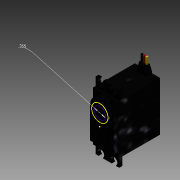
# Autodesk Inventor part: Tetrix 180 Servo
Saved by Autodesk Inventor 2013 (Build 170138000, 138)
## iProperties
Created: 2012-11-17
Part Number: Tetrix 180 Servo
Material: Generic
Document SubType Name: Modeling
Designer: niemitalo_dan
Density: 1 g/cm^3
Author: niemitalo_dan
Autodesk Inventor part; units mm, degrees
ref_plane "YZ Plane" through (0, 0, 0) normal (1, 0, 0) x (0, 1, 0)
ref_plane "XZ Plane" through (0, 0, 0) normal (0, 1, 0) x (-1, 0, 0)
sketch "Hole Pattern 4" plane through (0, 0, 0) normal (0, 0, 1) x (1, 0, 0)
  circle A0 centre (-145.7144, 104.3642) radius 4
  circle A1 centre (-145.7144, 104.3642) radius 8 construction
  circle A2 centre (-145.7144, 112.3642) radius 1.85
  circle A3 centre (-145.7144, 96.3642) radius 1.85
  circle A4 centre (-153.7144, 104.3642) radius 1.85
  circle A5 centre (-137.7144, 104.3642) radius 1.85
  circle A6 centre (-145.7144, 120.3642) radius 4
  circle A7 centre (-145.7144, 88.3642) radius 4
  point P0 (-145.7144, 107.7928)
  dimension "d140" = 16
  dimension "d141" = 3.7
  dimension "d142" = 16
  dimension "d143" = 16
  dimension "d144" = 8
  measures "d140" diameter of A1
  measures "d141" diameter of A2
  measures "d142" distance of A6.centre A0.centre
  measures "d143" distance of A7.centre A0.centre
  measures "d144" diameter of A0
sketch "Sketch1" plane through (0, 0, 0) normal (0, 0, 1) x (1, 0, 0)
  line L0 (-9.9314, 19.3675) -> (9.9314, 19.3675)
  line L1 (9.9314, 19.3675) -> (9.9314, -19.3675)
  line L2 (9.9314, -19.3675) -> (-9.9314, -19.3675)
  line L3 (-9.9314, -19.3675) -> (-9.9314, 19.3675)
  point P0 (0, 0)
  point P1 (-9.9314, 0)
  point P2 (0, 19.3675)
  dimension "d0" = 19.8628
  dimension "d1" = 38.735
  constraints: 8 end point, 2 midpoint, 2 parallel, 1 horizontal, 1 horizontal alignment, 1 perpendicular, 1 vertical alignment
  measures "d0" distance of L1.end L2.end
  measures "d1" distance of L0.end L1.end
extrude "Extrusion1" add sketch "Sketch1" along normal blind 33.147
sketch "Sketch2" plane through (0, 0, 33.147) normal (0, 0, 1) x (1, 0, 0)
  line L0 (9.9314, 19.3675) -> (-9.9314, 19.3675) projected
  line L1 (-9.9314, 19.3675) -> (-9.9314, -19.3675) projected
  line L2 (-9.9314, -19.3675) -> (9.9314, -19.3675) projected
  line L3 (-9.2964, 18.7325) -> (9.2964, 18.7325)
  line L4 (9.2964, 18.7325) -> (9.2964, -15.0495)
  line L5 (9.2964, -15.0495) -> (-9.2964, -15.0495)
  line L6 (-9.2964, -15.0495) -> (-9.2964, 18.7325)
  arc A0 (-3.6998, -15.0495) -> (3.6998, -15.0495) centre (0, -10.9617) ccw
  point P0 (0, 0)
  point P1 (0, 18.7325)
  dimension "d4" = 0.635
  dimension "d5" = 0.635
  dimension "d6" = 4.318
  constraints: 8 end point, 2 parallel, 2 point on circle, 2 point on line, 2 vertical alignment, 1 centre point, 1 horizontal, 1 midpoint, 1 perpendicular
  measures "d4" distance between parallel lines of L0 L3
  measures "d5" distance between parallel lines of L1 L6
  measures "d6" distance between parallel lines of L2 L5
extrude "Extrusion2" add sketch "Sketch2" along normal blind 2.794 contours L3 L4 L5 L6
sketch "Sketch3" plane through (0, 0, 35.941) normal (0, 0, 1) x (1, 0, 0)
  circle A0 centre (0, 9.4361) radius 6.4516
  line L0 (9.9314, 19.3675) -> (-9.9314, 19.3675) projected
  point P0 (0, 0)
  dimension "d9" = 12.9032
  dimension "d11" = 9.9314
  constraints: 1 centre point, 1 vertical alignment
  measures "d9" diameter of A0
  measures "d11" distance from line of L0 A0.centre
extrude "Extrusion3" add sketch "Sketch3" along normal blind 1.778
fillet "Fillet1" radius 9.2964 2 edges at (9.2964, 18.7325, 34.544) (-9.2964, 18.7325, 34.544)
ref_plane "Work Plane1" through (0, 0, 29.083) normal (0, 0, 1) x (1, 0, 0)
sketch "Sketch4" plane through (0, 0, 29.083) normal (0, 0, 1) x (1, 0, 0)
  line L0 (9.9314, 19.3675) -> (9.9314, -19.3675) projected
  line L1 (9.9314, -19.3675) -> (-9.9314, -19.3675) projected
  line L2 (-9.9314, -19.3675) -> (-9.9314, 19.3675) projected
  line L3 (-9.9314, 19.3675) -> (9.9314, 19.3675) projected
  line L4 (-9.3599, 19.3675) -> (9.3599, 19.3675)
  line L5 (9.3599, 19.3675) -> (9.3599, 26.4795)
  line L6 (-9.3599, 26.4795) -> (-9.3599, 19.3675)
  circle A0 centre (-5.1689, 23.9395) radius 2.667
  circle A1 centre (5.1689, 23.9395) radius 2.667
  line L7 (-5.9821, 26.4795) -> (-9.3599, 26.4795)
  line L8 (9.3599, 26.4795) -> (5.9821, 26.4795)
  line L9 (4.3557, 26.4795) -> (-4.3557, 26.4795)
  point P0 (0, 0)
  point P1 (0, 26.4795)
  dimension "d16" = 18.7198
  dimension "d18" = 7.112
  dimension "d20" = 5.334
  dimension "d21" = 4.191
  dimension "d22" = 4.191
  constraints: 12 end point, 4 parallel, 4 point on circle, 2 centre point, 1 equal radius, 1 horizontal, 1 horizontal alignment, 1 midpoint, 1 perpendicular, 1 point on line, 1 vertical alignment
  measures "d16" distance of L5.end L6.start
  measures "d18" distance of L6.start L4.start
  measures "d20" diameter of A0
  measures "d21" distance from line of L6 A0.centre
  measures "d22" distance from line of L5 A1.centre
extrude "Extrusion4" add sketch "Sketch4" along normal blind 2.54 contours L3 L6 L7 A0 L9 A1 L8 L5
fillet "Fillet2" radius 0.254 4 edges at (-5.9821, 26.4795, 30.353) (-4.3557, 26.4795, 30.353) (4.3557, 26.4795, 30.353) (5.9821, 26.4795, 30.353)
mirror "Mirror1" about plane through (0, 0, 0) normal (0, 1, 0) of "Extrusion4", "Fillet2"
sketch "Sketch5" plane through (-9.9314, 19.3675, 0) normal (0, 1, 0) x (1, 0, 0)
  line L0 (0, 0) -> (19.8628, 0) projected
  line L1 (6.1214, -0.254) -> (13.7414, -0.254)
  line L2 (13.7414, -0.254) -> (13.7414, -4.572)
  line L3 (13.7414, -4.572) -> (6.1214, -4.572)
  line L4 (6.1214, -4.572) -> (6.1214, -0.254)
  point P0 (9.9314, 0)
  point P1 (9.9314, -0.254)
  point P2 (9.9314, 0)
  dimension "d26" = 7.62
  dimension "d27" = 4.318
  dimension "d28" = 0.254
  constraints: 8 end point, 2 midpoint, 2 parallel, 1 horizontal, 1 perpendicular, 1 vertical alignment
  measures "d26" distance of L2.end L3.end
  measures "d27" distance of L1.end L2.end
  measures "d28" distance between parallel lines of L0 L1
extrude "Extrusion5" add sketch "Sketch5" along normal blind 1.5875
sketch "Sketch6" plane through (-9.9314, 20.955, 0) normal (0, 1, 0) x (1, 0, 0)
  line L0 (13.7414, -0.254) -> (6.1214, -0.254) projected
  line L1 (6.1214, -0.254) -> (6.1214, -4.572) projected
  line L2 (6.1214, -4.572) -> (13.7414, -4.572) projected
  line L3 (13.7414, -4.572) -> (13.7414, -0.254) projected
  point P0 (9.9314, 0)
extrude "Extrusion6" add sketch "Sketch6" along normal blind 5.08 draft -10
sketch "Sketch7" plane through (-9.9314, 26.035, 0) normal (0, 1, 0) x (1, 0, 0)
  circle A0 centre (9.9314, -2.413) radius 0.7937
  point P0 (9.9314, 0)
  dimension "d33" = 1.5875
  constraints: 1 centre point
  measures "d33" diameter of A0
extrude "Extrusion7" add sketch "Sketch7" along normal blind 5.08 separate body
sketch "Sketch8" plane through (-9.9314, 26.035, 0) normal (0, 1, 0) x (1, 0, 0)
  line L0 (7.0171, -3.6763) -> (7.0171, -1.1497) projected
  circle A0 centre (8.0331, -2.413) radius 0.7937
  point P0 (9.9314, 0)
  dimension "d36" = 1.5875
  dimension "d37" = 1.016
  constraints: 1 centre point
  measures "d36" diameter of A0
  measures "d37" distance from line of L0 A0.centre
extrude "Extrusion8" add sketch "Sketch8" along normal blind 5.08 bodies 1
sketch "Sketch9" plane through (-9.9314, 26.035, 0) normal (0, 1, 0) x (1, 0, 0)
  line L0 (12.8457, -1.1497) -> (12.8457, -3.6763) projected
  circle A0 centre (11.8297, -2.413) radius 0.7938
  point P0 (9.9314, 0)
  dimension "d40" = 1.5875
  dimension "d41" = 1.016
  constraints: 1 centre point
  measures "d40" diameter of A0
  measures "d41" distance from line of L0 A0.centre
extrude "Extrusion9" add sketch "Sketch9" along normal blind 5.08 separate body
sketch "Sketch25" plane through (0, 9.4361, 37.719) normal (0, 0, 1) x (1, 0, 0)
  circle A0 centre (0, 0) radius 6.4516 projected
  circle A1 centre (0, 0) radius 4.5085
  point P0 (0, -9.4361)
  dimension "d145" = 9.017
  constraints: 1 centre point, 1 coincident
  measures "d145" diameter of A1
equation "\"d5\" = d4"
equation "\"d22\" = d21"
